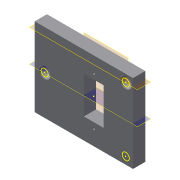
# Autodesk Inventor part: 05_Adapterplate_LG_CRD_8521B
Saved by Autodesk Inventor 2019 (Build 230136000, 136)
## iProperties
Created: 2019-06-12
Part Number: 05_Adapterplate_LG_CRD_8521B
Material: Generic
Document SubType Name: Modeling
Designer: diederichbenedict
Density: 1 g/cm^3
Appearance: Default
Author: diederichbenedict
Autodesk Inventor part; units mm, degrees
ref_plane "YZ Plane" through (0, 0, 0) normal (1, 0, 0) x (0, 1, 0)
ref_plane "XZ Plane" through (0, 0, 0) normal (0, 1, 0) x (-1, 0, 0)
ref_plane "XY Plane" through (0, 0, 0) normal (0, 0, 1) x (1, 0, 0)
ref_plane "Work Plane1" through (0, 0, 0) normal (0, 0, 1) x (1, 0, 0)
sketch "Sketch1" plane through (0, 0, 0) normal (0, 0, 1) x (1, 0, 0)
  circle A0 centre (0, -11.4) radius 0.5 construction
  circle A1 centre (0, 8.1) radius 0.5 construction
  circle A2 centre (0, -1.6) radius 3.9462 construction
  line L0 (8.2, 14.1) -> (-8.2, 14.1) construction
  line L1 (-8.2, 14.1) -> (-8.2, -14.1) construction
  line L2 (-8.2, -14.1) -> (8.2, -14.1) construction
  line L3 (8.2, -14.1) -> (8.2, 14.1) construction
  line L4 (-4, -9.1) -> (4, -9.1)
  line L5 (4, -9.1) -> (4, 5.9)
  line L6 (4, 5.9) -> (-4, 5.9)
  line L7 (-4, 5.9) -> (-4, -9.1)
  line L8 (-4, -9.1) -> (4, 5.9) construction
  line L9 (4, -9.1) -> (-4, 5.9) construction
  circle A3 centre (13, 11.4) radius 1.45 construction
  circle A4 centre (13, -14.6) radius 1.45 construction
  circle A5 centre (-20, -1.6) radius 1.45 construction
  line L10 (16, -17.6) -> (16, 14.4) construction
  line L11 (16, 14.4) -> (-16, 14.4) construction
  line L12 (-16, -17.6) -> (16, -17.6) construction
  line L13 (16, 14.4) -> (-24, 14.4)
  line L14 (-24, 14.4) -> (-24, -17.6)
  line L15 (-24, -17.6) -> (16, -17.6)
  line L16 (16, -17.6) -> (16, 14.4)
  circle A6 centre (0, 8.1) radius 0.5
  circle A7 centre (0, -11.4) radius 0.5
  point P0 (0, 0)
extrude "Extrusion1" add sketch "Sketch1" along normal blind 5
ref_plane "Work Plane2" through (-24, -1.6, 0) normal (0, -1, 0) x (1, 0, 0)
sketch "Sketch2" plane through (-24, -1.6, 0) normal (0, -1, 0) x (1, 0, 0)
  line L0 (1, 9) -> (1, 5)
  line L1 (7, 9) -> (7, 5)
  circle A0 centre (4, 4) radius 2.55
  line L2 (4, 6.55) -> (4, 1.45)
  point P0 (24, 0)
  dimension "d6" = 5.1
  dimension "d7" = 3
  dimension "d8" = 1
  constraints: 6 end point, 3 vertical, 2 point on circle, 1 centre point, 4 other
  measures "d6" diameter of A0
  measures "d7" distance from line of A0.centre L0
  measures "d8" vertical distance of L0.end A0.centre
revolve "Revolution1" cut sketch "Sketch2" angle 360 about axis through (-20, -1.6, 6.55) along (0, 0, -1) picked at (3.097, 3.5418) contours L2 A0
sketch "Sketch3" plane through (0, 0, 5) normal (0, 0, 1) x (1, 0, 0)
  circle A0 centre (13, -14.6) radius 1.45 projected
  circle A1 centre (13, 11.4) radius 1.45 projected
  circle A2 centre (-20, -1.6) radius 1.45 projected
  point P0 (0, 0)
ref_plane "Work Plane3" through (13, 11.4, 5) normal (0, 1, 0) x (1, 0, 0)
sketch "Sketch4" plane through (13, 11.4, 5) normal (0, 1, 0) x (1, 0, 0)
  circle A0 centre (0, 1) radius 2.55
  line L0 (-37, 0) -> (3, 0) projected
  line L1 (0, -4) -> (0, 0) projected
  line L2 (0, 0) -> (0, 3.55)
  line L3 (0, -1.55) -> (0, 0)
  point P0 (-13, 5)
  dimension "d10" = 5.1
  dimension "d11" = 1
  dimension "d12" = 0
  constraints: 4 end point, 2 point on circle, 1 centre point, 1 collinear, 1 point on line, 1 vertical
  measures "d10" diameter of A0
  measures "d11" distance from line of L0 A0.centre
  measures "d12" distance from line of A0.centre L1
revolve "Revolution2" cut sketch "Sketch4" angle 360 about axis through (13, 11.4, 5) along (0, 0, -1) picked at (-0.2076, 2.3409) picked at (-1.4654, -0.1719) contours L2 L0 A0 | L0 L1 A0
ref_plane "Work Plane4" through (13, -14.6, 5) normal (0, -1, 0) x (1, 0, 0)
sketch "Sketch5" plane through (13, -14.6, 5) normal (0, -1, 0) x (1, 0, 0)
  line L0 (0, 4) -> (0, 0) projected
  arc A0 (0, -3.55) -> (0, 1.55) centre (0, -1) ccw
  line L1 (0, 1.55) -> (0, -3.55)
  arc A1 (-2.3457, 0) -> (2.3457, 0) centre (0, -1) ccw projected
  point P0 (-13, -5)
  dimension "d14" = 5.1
  dimension "d15" = 1
  constraints: 3 point on circle, 2 end point, 1 centre point, 1 point on line, 1 vertical
  measures "d14" diameter of A0
  measures "d15" distance of L0.end A0.centre
revolve "Revolution3" cut sketch "Sketch5" angle 360 about axis through (13, -14.6, 9) along (0, 0, -1)
body "Solid1"
